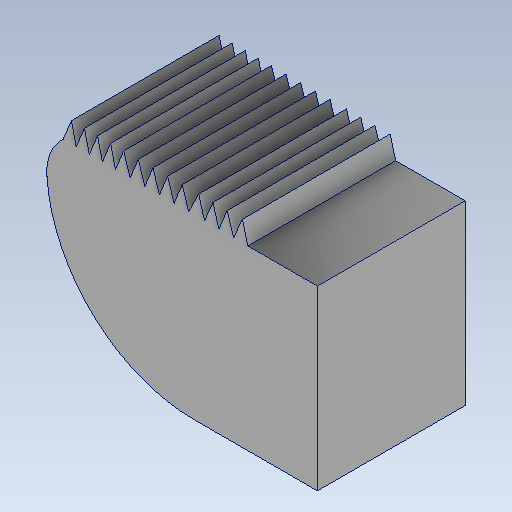
# Autodesk Inventor part: Finray_9_Kerbe_10deg_anschluss_erweitert_9_75 Nut
Saved by Autodesk Inventor 2025.2 (Build 292293000, 293)
## iProperties
Created: 2022-02-28
Part Number: Finray_9_Kerbe_10deg_anschluss_erweitert_9_75 Nut
Material: Generic
Document SubType Name: Modeling
Designer: richa
Density: 1 g/cm^3
Appearance: Aluminum - Flat
Author: richa
## iProperties of the stored document Maria_Greifer_3D-Druck.ipt
Created: 2024-11-10
Part Number: Maria_Greifer_3D-Druck
Material: Generisch
Document SubType Name: Modeling
Designer: maria
Density: 1 g/cm^3
Appearance: Vorgabe
Author: maria
Autodesk Inventor part; units mm, degrees
ref_plane "YZ Plane" through (0, 0, 0) normal (1, 0, 0) x (0, 1, 0)
ref_plane "XZ Plane" through (0, 0, 0) normal (0, 1, 0) x (-1, 0, 0)
ref_plane "XY Plane" through (0, 0, 0) normal (0, 0, 1) x (1, 0, 0)
sketch "Sketch5" plane through (0, 0, 0) normal (0, 0, 1) x (1, 0, 0)
  line L0 (27.5, -18) -> (0, -18)
  line L1 (0, -18) -> (0, 0)
  line L2 (27.5, -1.0645) -> (27.5, -18)
  line L3 (1.6866, 0) -> (2.5215, 2.0553)
  line L4 (2.5215, 2.0553) -> (3.0145, 0)
  line L5 (3.0145, 0) -> (3.8493, 2.0553)
  line L6 (3.8493, 2.0553) -> (4.3423, 0)
  line L7 (4.3423, 0) -> (5.1772, 2.0553)
  line L8 (5.1772, 2.0553) -> (5.6702, 0)
  line L9 (5.6702, 0) -> (6.505, 2.0553)
  line L10 (6.505, 2.0553) -> (6.998, 0)
  line L11 (6.998, 0) -> (7.8329, 2.0553)
  line L12 (7.8329, 2.0553) -> (8.4844, 0)
  line L13 (8.4844, 0) -> (9.3192, 2.0553)
  line L14 (9.3192, 2.0553) -> (9.9707, 0)
  line L15 (9.9707, 0) -> (10.8056, 2.0553)
  line L16 (10.8056, 2.0553) -> (11.4571, 0)
  line L17 (11.4571, 0) -> (12.292, 2.0553)
  line L18 (12.292, 2.0553) -> (12.9435, 0)
  line L19 (12.9435, 0) -> (13.7783, 2.0553)
  line L20 (13.7783, 2.0553) -> (14.4298, 0)
  line L21 (14.4298, 0) -> (15.4488, 2.0563)
  line L22 (15.4488, 2.0563) -> (16.0375, 0.0047)
  line L23 (16.0375, 0.0047) -> (16.8992, 2.0553)
  line L24 (16.8992, 2.0553) -> (17.489, 0)
  line L25 (0, 0) -> (1.6866, 0)
  line L26 (0, 0) -> (1.6866, 0)
  line L27 (17.489, 0) -> (18.3372, 2.0553)
  line L28 (18.3372, 2.0553) -> (18.989, -0.0011)
  line L29 (27.5, -0.0004) -> (27.5, -1.0645)
  line L30 (18.989, -0.0011) -> (19.8773, 2.0553)
  line L31 (19.8773, 2.0553) -> (20.4405, -0.0004)
  line L32 (15.4483, 2.0553) -> (15.4491, 2.0553)
  line L33 (18.9887, 0) -> (18.9895, 0)
  line L34 (20.4405, -0.0004) -> (27.5, -0.0004)
  point P0 (20.4491, -0.0317)
  dimension "d97" = 18
  dimension "d106" = 27.5
  constraints: 73 end point, 9 parallel, 5 point on line, 4 horizontal, 1 perpendicular
  measures "d97" distance of L0.end L1.end
  measures "d106" distance of L0.start L0.end
extrude "Extrusion2" add sketch "Sketch5" along normal blind 15
fillet "Fillet2" radius 15 1 edges at (0, -18, 7.5)
fillet "Rundung3" radius 5 1 edges at (0, 0, 7.5)
equation "\"l1\" = 8"
body "Solid2"
